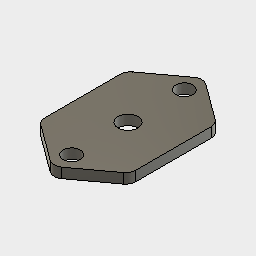
Bolt_Guide_Plate (Autodesk Fusion 360 design; units mm, degrees)
Autodesk Fusion 360 part; units mm, degrees
sketch "Plate" plane through (0, 0, 0) normal (0, 1, 0) x (1, 0, 0) in component "Plate"
  line L0 (0, 0) -> (-22.8, 0)
  line L1 (-22.8, 0) -> (-22.8, 21.5)
  line L2 (-22.8, 21.5) -> (0, 38.25)
  line L3 (0, -20) -> (0, -2.5)
  line L4 (2.5, 0) -> (20, 0)
  line L5 (22.8, 21.5) -> (0, 38.25)
  line L6 (22.8, 0) -> (22.8, 21.5)
  line L7 (0, 0) -> (22.8, 0)
  point P0 (0, 38.25)
  dimension "d2" = 22.8
  dimension "d41" = 21.5
  dimension "d42" = 38.25
  dimension "d83" = 0
  dimension "d84" = 0
  dimension "d85" = 0
  dimension "d86" = 0
  measures "d2" distance of L0.start L0.end
  measures "d41" distance of L0 L1.end
  measures "d42" distance of P0 L0.start
extrude "Extrude1" add sketch "Plate" along normal blind 5 makes body 1 in component "Plate"
fillet "Fillet3" radius 5 1 edges at (0, 2.5, -38.25) on bodies 1 in component "Plate"
fillet "Fillet4" radius 5 1 edges at (-22.8, 2.5, -21.5) on bodies 1 in component "Plate"
fillet "Fillet5" radius 5 1 edges at (22.8, 2.5, -21.5) on bodies 1 in component "Plate"
hole "Hole1" at (0, 5, -28.25) direction (0, -1, 0) diameter 8.5 end through all bodies 1 in component "Plate"
mirror "Mirror1" about plane through (0, 0, 0) normal (0, 0, 1) of bodies 1 makes body 2 in component "Plate"
combine "Combine1" operation add target body 1 tool bodies 2 in component "Plate"
hole "Hole1'" at (0, 5, 0) direction (0, -1, 0) diameter 10 end through all bodies 1 in component "Plate"
component "Plate" placed x (1, 0, 0) y (0, 1, 0) z (0, 0, 1) at (0, 0, 0)
